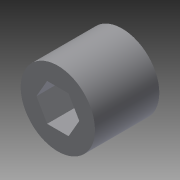
# Autodesk Inventor part: 3dprintedspacer
Saved by Autodesk Inventor 2014 SP1 (Build 180222100, 222)
## iProperties
Created: 2014-01-30
Part Number: 3dprintedspacer
Material: Generic
Document SubType Name: Modeling
Designer: Arpan
Density: 1 g/cm^3
Appearance: Default
Author: Arpan
Autodesk Inventor part; units mm, degrees
ref_plane "YZ Plane" through (0, 0, 0) normal (1, 0, 0) x (0, 1, 0)
ref_plane "XZ Plane" through (0, 0, 0) normal (0, 1, 0) x (-1, 0, 0)
ref_plane "XY Plane" through (0, 0, 0) normal (0, 0, 1) x (1, 0, 0)
sketch "Sketch1" plane through (0, 0, 0) normal (0, 0, 1) x (1, 0, 0)
  line L0 (3.6662, 6.35) -> (7.3323, 0)
  line L1 (7.3323, 0) -> (3.6662, -6.35)
  line L2 (3.6662, -6.35) -> (-3.6662, -6.35)
  line L3 (-3.6662, -6.35) -> (-7.3323, 0)
  line L4 (-7.3323, 0) -> (-3.6662, 6.35)
  line L5 (-3.6662, 6.35) -> (3.6662, 6.35)
  circle A0 centre (0, 0) radius 12.7
  dimension "d0" = 6.35
  dimension "d1" = 25.4
  constraints: 12 end point, 2 coincident, 1 centre point, 13 other
  measures "d0" distance from line of L5 point (0, 0)
  measures "d1" diameter of A0
extrude "Extrusion1" add sketch "Sketch1" along normal blind 21.9964
body "Solid1"
